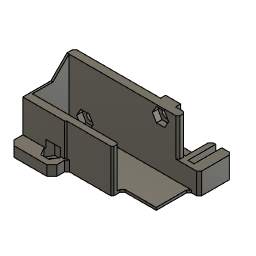
Batterihållare v6 (Autodesk Fusion 360 design; units mm, degrees)
Autodesk Fusion 360 part; units mm, degrees
sketch "Sketch1" plane through (0, 0, 0) normal (0, 1, 0) x (1, 0, 0)
  line L0 (-12, -5) -> (5, -5)
  line L1 (0, 0) -> (0, -5) construction
  line L2 (0, 0) -> (-12, 0) construction
  line L3 (5, -5) -> (5, 1)
  line L4 (5, 1) -> (23, 1)
  line L5 (23, 5) -> (36.4, 5)
  line L6 (36.4, 5) -> (36.4, 20)
  line L7 (23, 5) -> (23, 1)
  line L8 (36.4, 20) -> (34, 20)
  line L9 (34, 20) -> (34, 31)
  line L10 (34, 31) -> (5, 31)
  line L11 (5, 31) -> (5, 37)
  line L12 (5, 37) -> (-5, 37)
  line L13 (-5, 37) -> (-5, 31)
  line L14 (-12, -5) -> (-12, 31)
  line L15 (-12, 31) -> (-5, 31)
  circle A0 centre (0, 0) radius 1.7
  line L16 (0, 0) -> (0, 32.5) construction
  circle A1 centre (0, 32.5) radius 1.7
  line L17 (5, 1) -> (5, 3.5)
  line L18 (5, 3.5) -> (-12, 3.5)
  line L19 (5, 31) -> (5, 28.9)
  line L20 (5, 28.9) -> (-5, 28.9)
  line L21 (-5, 31) -> (-5, 28.9)
  line L22 (-12, 18) -> (32, 18)
  line L23 (5, 3.5) -> (23, 3.5)
  line L24 (-12, 21) -> (32, 21)
  line L25 (32, 21) -> (32, 18)
  line L26 (5, 0.5) -> (-12, 0.5)
  line L27 (-11.2, 18) -> (-11.2, 3.5)
  dimension "d1" = 5
  dimension "d2" = 12
  dimension "d3" = 5
  dimension "d10" = 1
  dimension "d12" = 5
  dimension "d13" = 36.4
  dimension "d14" = 20
  dimension "d16" = 23
  dimension "d17" = 34
  dimension "d18" = 31
  dimension "d19" = 5
  dimension "d20" = 37
  dimension "d22" = 5
  dimension "d23" = 31
  dimension "d26" = 3.4
  dimension "d27" = 32.5
  dimension "d28" = 3.5
  dimension "d31" = 28.9
  dimension "d44" = 18
  dimension "d45" = 3
  dimension "d53" = 44
  dimension "d54" = 3
  dimension "d57" = 0.8
  constraint horizontal L0
  constraint coincident L1.start L2.start
  constraint coincident L0 L1.end
  constraint perpendicular L0 L1
  constraint perpendicular L0 L3
  constraint perpendicular L3 L4
  constraint perpendicular L5 L6
  constraint perpendicular L5 L7
  constraint perpendicular L4 L7
  constraint perpendicular L6 L8
  constraint perpendicular L8 L9
  constraint perpendicular L1 L10
  constraint perpendicular L10 L11
  constraint perpendicular L11 L12
  constraint perpendicular L12 L13
  constraint perpendicular L0 L14
  constraint perpendicular L13 L15
  constraint coincident L2.end L14
  constraint perpendicular L2 L14
  constraint perpendicular L2 L16
  constraint coincident L16.end A1.centre
  constraint equal A0 A1
  constraint perpendicular L4 L17
  constraint coincident L14 L18.end
  constraint perpendicular L14 L18
  constraint perpendicular L10 L19
  constraint perpendicular L19 L20
  constraint perpendicular L20 L21
  constraint coincident L14 L22.start
  constraint coincident L7 L23.end
  constraint perpendicular L7 L23
  constraint coincident L14 L24.start
  constraint perpendicular L24 L25
  constraint coincident L3 L26.start
  constraint coincident L14 L26.end
  constraint perpendicular L14 L26
  constraint coincident L22 L27.start
  constraint coincident L18 L27.end
  constraint perpendicular L18 L27
  measures "d1" distance of L1.start L1.end
  measures "d2" distance of L1.start L2.end
  measures "d3" distance of L0.end L1
  measures "d10" vertical distance of L1.start L3.end
  measures "d12" vertical distance of L1.start L5.start
  measures "d13" horizontal distance of L1.start L5.end
  measures "d14" vertical distance of L1.start L6.end
  measures "d16" distance of L1.start L7
  measures "d17" horizontal distance of L1.start L8.end
  measures "d18" vertical distance of L1.start L9.end
  measures "d19" horizontal distance of L1.start L10.end
  measures "d20" vertical distance of L1.start L11.end
  measures "d22" horizontal distance of L1.start L12.end
  measures "d23" vertical distance of L1.start L13.end
  measures "d26" diameter of A0
  measures "d27" distance of L1.start L16.end
  measures "d28" distance of L1.start L18
  measures "d31" distance of L1.start L20
  measures "d44" distance of L1.start L22
  measures "d45" distance of L22 L24
  measures "d53" distance of L14 L25
  measures "d54" distance of L18 L26
  measures "d57" distance of L14 L27
extrude "Extrude1" add sketch "Sketch1" along normal blind 1 contours L14 L18 L22 L27 | L4 L7 L17 L23 | L14 L22 L24 L25 | L5 L6 L7 L8 L9 L10 L14 L15 L18 L19 L20 L21 L22 L23 L24 L25 L27 makes body 1
extrude "Extrude2" add sketch "Sketch1" along normal blind 4 contours L0 L3 L14 A0 L26 | L3 L14 A0 L17 L18 L26 | A0 L26 | A0 L26 bodies 1
extrude "Extrude14" add sketch "Sketch1" along normal blind 2 contours L11 L12 L13 L19 L20 L21 bodies 1
sketch "Sketch2" plane through (0, 1, 0) normal (0, 1, 0) x (-1, 0, 0)
  line L0 (-36.4, -5) -> (-36.4, -20)
  line L1 (-36.4, -20) -> (-34, -20)
  line L2 (-34, -20) -> (-34, -31)
  line L3 (-34, -31) -> (-5, -31)
  line L4 (5, -31) -> (12, -31)
  line L5 (12, -31) -> (12, -3.5)
  line L6 (-34, -20) -> (-34, -31)
  line L7 (-36.4, -20) -> (-34, -20)
  line L8 (-36.4, -20) -> (-36.4, -31)
  line L9 (-36.4, -31) -> (-40.4, -31)
  line L10 (-40.4, -31) -> (-40.4, -16)
  line L11 (-40.4, -16) -> (-36.4, -16)
  line L12 (-36.4, -16) -> (-32, -16)
  line L13 (-32, -16) -> (-32, -31)
  line L14 (-37, -19.4) -> (-37, -31)
  line L15 (-37, -19.4) -> (-33.4, -19.4)
  line L16 (-33.4, -19.4) -> (-33.4, -31)
  line L17 (-5, -1) -> (-23, -1)
  line L18 (-23, -1) -> (-23, -5)
  line L19 (-23, -5) -> (-36.4, -5)
  line L20 (12, -3.5) -> (-5, -3.5)
  line L21 (-5, -3.5) -> (-5, -1)
  line L22 (-34, -20) -> (-34, -31)
  line L23 (-5, -31) -> (-5, -28.9)
  line L24 (-5, -28.9) -> (5, -28.9)
  line L25 (5, -28.9) -> (5, -31)
  dimension "d33" = 4
  dimension "d35" = 4
  dimension "d43" = 0.6
  dimension "d67" = 2
  constraint perpendicular L8 L9
  constraint coincident L0 L11.end
  constraint perpendicular L0 L11
  constraint perpendicular L9 L10
  constraint perpendicular L0 L12
  constraint perpendicular L12 L13
  constraint coincident L0.end L1.start
  constraint collinear L3 L9
  constraint coincident L3 L13.end
  measures "d33" distance of L8.end L9.end
  measures "d35" distance of L0.end L11
  measures "d67" distance of L13 L22
extrude "Extrude3" add sketch "Sketch2" along normal blind 7.5 and the other way blind -5 separate body contours L0 L3 L12 L13 L15 L16 | L0 L9 L10 L11 L14 L15 | L0 L1 L2 L3 L6 L7 L15 L16 L22 | L0 L8 L9 L14 L15 makes body 2
extrude "Extrude4" add sketch "Sketch2" along normal blind 7.5 and the other way blind 1 contours L0 L3 L12 L13 L15 L16 | L0 L9 L10 L11 L14 L15 bodies 2 1
extrude "Extrude5" cut 1 faces at (33.6, 1, -23.4667) along direction (0, -1, 0) blind 1 on bodies 2 bodies 2
extrude "Extrude6" add sketch "Sketch1" along normal blind 23.4 contours L14 L22 L24 L25 bodies 2
extrude "Extrude15" add sketch "Sketch1" along normal blind 17 contours L3 L14 A0 L17 L18 L26 | L14 L18 L22 L27 | A0 L26 | L4 L7 L17 L23 picked at (-0.2599, 1.2317) bodies 2
chamfer "Chamfer14" distance 6.4 angle 45 1 edges at (-11.6, 17, -18) on bodies 2
extrude "Extrude8" cut sketch "Sketch1" along normal blind 6 contours A0 L26 | A0 L26 bodies 2
extrude "Extrude9" cut 1 faces at (36.2667, 6, -16) along direction (0, 0, -1) blind 2 on bodies 2 bodies 2
sketch "Sketch3" plane through (0, 4, 0) normal (0, 1, 0) x (-1, 0, 0)
  line L0 (1.5877, -29.75) -> (-1.5877, -29.75)
  line L1 (-1.5877, -29.75) -> (-3.1754, -32.5)
  line L2 (-3.1754, -32.5) -> (-1.5877, -35.25)
  line L3 (-1.5877, -35.25) -> (1.5877, -35.25)
  line L4 (1.5877, -35.25) -> (3.1754, -32.5)
  line L5 (3.1754, -32.5) -> (1.5877, -29.75)
  line L6 (1.5877, 2.75) -> (-1.5877, 2.75)
  line L7 (-1.5877, 2.75) -> (-3.1754, 0)
  line L8 (-3.1754, 0) -> (-1.5877, -2.75)
  line L9 (-1.5877, -2.75) -> (1.5877, -2.75)
  line L10 (1.5877, -2.75) -> (3.1754, 0)
  line L11 (3.1754, 0) -> (1.5877, 2.75)
  arc A0 (1.6248, -0.5) -> (-1.6248, -0.5) centre (0, 0) ccw
  line L12 (12, -0.5) -> (12, 5)
  line L13 (12, 5) -> (-5, 5)
  line L14 (-5, 5) -> (-5, -0.5)
  line L15 (1.6248, -0.5) -> (12, -0.5)
  line L16 (-5, -0.5) -> (-1.6248, -0.5)
  circle A1 centre (0, -32.5) radius 1.7
  point P0 (0, -32.5)
  dimension "d62" = 5.5
  constraint coincident A0.centre origin
  constraint equal L5 L11
  constraint horizontal L3
  constraint horizontal L6
  constraint coincident P0 A1.centre
  measures "d62" distance of L2 L5
extrude "Extrude10" cut sketch "Sketch3" along normal mid plane 6 contours L0 L1 L2 L3 L4 L5 | L6 L7 L8 L10 L11 A0 L15 L16 | L8 L9 L10 A0 L15 L16 | A1 bodies 2
sketch "Sketch4" plane through (0, 0, -21) normal (0, 0, -1) x (-1, 0, 0)
  line L0 (-32, 8.5) -> (-32, 1)
  line L1 (-32, 1) -> (12, 1)
  line L2 (12, 1) -> (12, 23.4)
  line L3 (12, 23.4) -> (-32, 23.4)
  line L4 (-32, 23.4) -> (-32, 8.5)
  line L5 (-31.6, 22.4) -> (11.4, 22.4) construction
  line L6 (11.4, 22.4) -> (11.4, 1.4) construction
  line L7 (11.4, 1.4) -> (-31.6, 1.4) construction
  line L8 (-31.6, 1.4) -> (-31.6, 22.4) construction
  circle A0 centre (-25.1, 19.9) radius 1.5
  circle A1 centre (4.9, 3.9) radius 1.5
  circle A2 centre (-25.1, 19.9) radius 3 construction
  circle A3 centre (4.9, 3.9) radius 3 construction
  line L9 (-32, 1) -> (-32, 8.5) construction
  line L10 (12, 1) -> (-32, 1) construction
  line L11 (-23.4834, 22.7) -> (-26.7166, 22.7)
  line L12 (-26.7166, 22.7) -> (-28.3332, 19.9)
  line L13 (-28.3332, 19.9) -> (-26.7166, 17.1)
  line L14 (-26.7166, 17.1) -> (-23.4834, 17.1)
  line L15 (-23.4834, 17.1) -> (-21.8668, 19.9)
  line L16 (-21.8668, 19.9) -> (-23.4834, 22.7)
  line L17 (6.5454, 6.75) -> (3.2546, 6.75)
  line L18 (3.2546, 6.75) -> (1.6091, 3.9)
  line L19 (1.6091, 3.9) -> (3.2546, 1.05)
  line L20 (3.2546, 1.05) -> (6.5454, 1.05)
  line L21 (6.5454, 1.05) -> (8.1909, 3.9)
  line L22 (8.1909, 3.9) -> (6.5454, 6.75)
  line L23 (1.9, 1) -> (7.9, 1)
  line L24 (7.9, 1) -> (7.9, 6.8)
  line L25 (7.9, 6.8) -> (1.9, 6.8)
  line L26 (1.9, 6.8) -> (1.9, 1)
  line L27 (1.9, 1) -> (7.9, 6.8) construction
  line L28 (7.9, 1) -> (1.9, 6.8) construction
  line L29 (-22.1, 23.4) -> (-28.1, 23.4)
  line L30 (-28.1, 23.4) -> (-28.1, 16.4)
  line L31 (-28.1, 16.4) -> (-22.1, 16.4)
  line L32 (-22.1, 16.4) -> (-22.1, 23.4)
  line L33 (-22.1, 23.4) -> (-28.1, 16.4) construction
  line L34 (-28.1, 23.4) -> (-22.1, 16.4) construction
  point P0 (-25.1, 19.9)
  point P1 (4.9, 3.9)
  point P2 (4.9, 3.9)
  point P3 (-25.1, 19.9)
  dimension "d65" = 21
  dimension "d66" = 43
  dimension "d70" = 6.5
  dimension "d71" = 6.5
  dimension "d72" = 6
  dimension "d73" = 0.4
  dimension "d74" = 0.4
  dimension "d75" = 3
  dimension "d76" = 5.6
  dimension "d77" = 5.7
  dimension "d92" = 6
  dimension "d96" = 2.5
  dimension "d97" = 2.5
  constraint horizontal L5
  constraint vertical L6
  constraint horizontal L7
  constraint vertical L8
  constraint concentric A0 A2
  constraint concentric A1 A3
  constraint equal A2 A3
  constraint equal A0 A1
  constraint coincident P3 P0
  constraint coincident P2 P1
  constraint horizontal L14
  constraint horizontal L17
  constraint horizontal L23
  constraint perpendicular L23 L24
  constraint parallel L23 L25
  constraint parallel L24 L26
  constraint coincident L27 P2
  constraint coincident L28 P2
  constraint horizontal L29
  constraint perpendicular L29 L30
  constraint parallel L29 L31
  constraint parallel L30 L32
  constraint coincident L33 P3
  constraint coincident L34 P3
  constraint equal L25 L29
  constraint collinear L3 L29
  constraint collinear L10 L23
  measures "d65" distance of L5.end L6.end
  measures "d66" distance of L5.start L5.end
  measures "d70" distance of L8 P3
  measures "d71" distance of L6 P2
  measures "d72" diameter of A2
  measures "d73" distance of L8 L9
  measures "d74" distance of L7 L10
  measures "d75" diameter of A0
  measures "d76" distance of L13 L16
  measures "d77" distance of L19 L22
  measures "d92" distance of L30 L32
  measures "d96" distance of L5 P3
  measures "d97" distance of L7 P2
extrude "Extrude13" add sketch "Sketch4" along normal blind 2 contours L1 L19 L20 L21 L23 L24 L26 | L3 L11 L12 L16 L29 L30 L32 | L17 L18 L19 L20 L21 L22 L24 L26 | L11 L12 L13 L14 L15 L16 L30 L32 | L17 L18 L22 L24 L25 L26 | L13 L14 L15 L30 L31 L32 bodies 2
extrude "Extrude12" cut sketch "Sketch4" along normal blind -0.8 and the other way blind 4 contours L17 L18 L19 L20 L21 L22 L24 L26 | L18 L19 L26 | L12 L13 L30 | L11 L12 L13 L14 L15 L16 L30 L32 | L21 L22 L24 | L15 L16 L32 bodies 2
extrude "Extrude11" cut sketch "Sketch4" against normal blind 5 contours A0 | A1 bodies 2
chamfer "Chamfer20" distance 2 angle 45 2 edges at (5, 2, 5) (-12, 2, 5) on bodies 2
chamfer "Chamfer19" distance 0.6 angle 45 2 edges at (23, 9, -3.5) (23, 8.5, -1) on bodies 2
chamfer "Chamfer16" distance 0.5 angle 45 1 edges at (5, 10.5, -0.5) on bodies 2
chamfer "Chamfer3" distance 2 angle 45 1 edges at (-12, 0.5, -31) on bodies 2
chamfer "Chamfer12" distance 2 angle 45 2 edges at (-5, 1, -37) (5, 1, -37) on bodies 2
chamfer "Chamfer5" distance 0.8 angle 45 3 edges at (32, 15.95, -21) (32, 15.95, -18) (-12, 12.2, -21) on bodies 2
chamfer "Chamfer6" distance 1 angle 45 3 edges at (5, 2, -1) (23, 0.5, -5) (36.4, 0.5, -18) on bodies 2
chamfer "Chamfer8" distance 1 angle 45 3 edges at (32, 4.75, -31) (40.4, 4.25, -31) (40.4, 4.25, -18) on bodies 2
chamfer "Chamfer10" distance 2 angle 45 1 edges at (25.1, 16.4, -21) on bodies 2
chamfer "Chamfer13" distance 2 angle 45 2 edges at (5, 0.5, -31) (-5, 0.5, -31) on bodies 2
chamfer "Chamfer17" distance 0.6 angle 45 3 edges at (37, 6, -25.2) (35.2, 6, -19.4) (33.4, 6, -25.2) on bodies 2
chamfer "Chamfer18" distance 2 angle 45 2 edges at (-5, 1.5, -28.9) (5, 1.5, -28.9) on bodies 2
equation "d36 = 6 mm - 1 mm + 2.5 mm"
equation "d38 = -6 mm + 1 mm"
equation "d40 = 6 mm - 1 mm + 2.5 mm"
equation "d44 = 18.5 mm - 0.5 mm"
equation "d50 = 23 mm + 0.4 mm"
equation "d104 = 16 mm + 1 mm"
named bodies: "Batterihållare"
